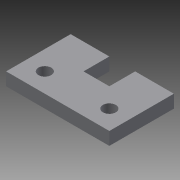
# Autodesk Inventor part: P1-2
Saved by Autodesk Inventor 2014 (Build 180170000, 170)
## iProperties
Created: 2017-02-06
Part Number: P1-2
Material: Generic
Document SubType Name: Modeling
Designer: mschaffel
Density: 1 g/cm^3
Appearance: Default
Author: mschaffel
Autodesk Inventor part; units mm, degrees
ref_plane "YZ Plane" through (0, 0, 0) normal (1, 0, 0) x (0, 1, 0)
ref_plane "XZ Plane" through (0, 0, 0) normal (0, 1, 0) x (-1, 0, 0)
ref_plane "XY Plane" through (0, 0, 0) normal (0, 0, 1) x (1, 0, 0)
sketch "Sketch1" plane through (0, 0, 0) normal (0, 1, 0) x (-1, 0, 0)
  line L0 (0, 0) -> (0, 63.5)
  line L1 (0, 63.5) -> (101.6, 63.5)
  line L2 (101.6, 63.5) -> (101.6, 0)
  line L3 (101.6, 0) -> (63.5, 0)
  line L4 (63.5, 0) -> (63.5, 25.4)
  line L5 (63.5, 25.4) -> (38.1, 25.4)
  line L6 (38.1, 25.4) -> (38.1, 0)
  line L7 (38.1, 0) -> (0, 0)
  circle A0 centre (19.05, 44.45) radius 6.35
  circle A1 centre (82.55, 44.45) radius 6.35
  dimension "d0" = 63.5
  dimension "d1" = 101.6
  dimension "d2" = 38.1
  dimension "d3" = 25.4
  dimension "d4" = 25.4
  dimension "d5" = 25.4
  dimension "d6" = 12.7
  dimension "d7" = 12.7
  constraints: 16 end point, 4 perpendicular, 3 parallel, 2 centre point, 1 vertical
  measures "d0" distance of L0.start L0.end
  measures "d1" distance of L0.end L1.end
  measures "d2" distance of L2.end L3.end
  measures "d3" distance of L3.end L4.end
  measures "d4" distance of L4.end L5.end
  measures "d5" distance of L5.end L6.end
  measures "d6" diameter of A0
  measures "d7" diameter of A1
extrude "Extrusion1" add sketch "Sketch1" along normal blind 12.7
body "Solid1"
